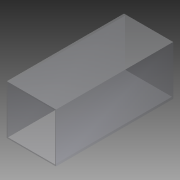
# Autodesk Inventor part: Placeholderbucket
Saved by Autodesk Inventor 2015 SP1 (Build 190203100, 203)
## iProperties
Created: 2014-11-21
Part Number: Placeholderbucket
Material: Polycarbonate, Clear
Document SubType Name: Modeling
Designer: sapatel
Density: 1.2 g/cm^3
Appearance: Polycarbonate - Clear
Author: sapatel
Autodesk Inventor part; units mm, degrees
ref_plane "YZ Plane" through (0, 0, 0) normal (1, 0, 0) x (0, 1, 0)
ref_plane "XZ Plane" through (0, 0, 0) normal (0, 1, 0) x (-1, 0, 0)
ref_plane "XY Plane" through (0, 0, 0) normal (0, 0, 1) x (1, 0, 0)
sketch "Sketch1" plane through (0, 0, 0) normal (0, 0, 1) x (1, 0, 0)
  line L0 (0, 0) -> (50.8, 0)
  line L1 (50.8, 0) -> (50.8, 50.8)
  line L2 (50.8, 50.8) -> (0, 50.8)
  line L3 (0, 50.8) -> (0, 0)
  line L4 (-1.27, 52.07) -> (52.07, 52.07)
  line L5 (52.07, 52.07) -> (52.07, -1.27)
  line L6 (52.07, -1.27) -> (-1.27, -1.27)
  line L7 (-1.27, -1.27) -> (-1.27, 52.07)
  dimension "d0" = 50.8
  dimension "d1" = 50.8
  dimension "d2" = 1.27
  constraints: 16 end point, 4 parallel, 2 perpendicular, 1 horizontal, 3 other
  measures "d0" distance of L2.end L1.end
  measures "d1" distance of L1.end L0.end
  measures "d2" distance between parallel lines of L2 L4
extrude "Extrusion1" add sketch "Sketch1" along normal blind 127
body "Solid1"
